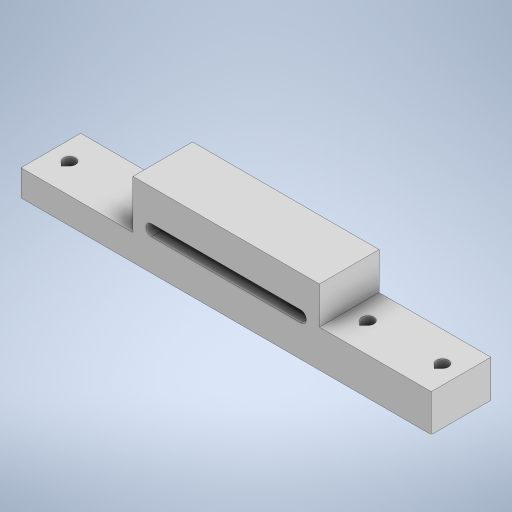
# Autodesk Inventor part: middle_hole
Saved by Autodesk Inventor 2023.1 (Build 271208000, 208)
## iProperties
Created: 2023-11-20
Part Number: middle_hole
Material: Všeobecné
Document SubType Name: Modeling
Designer: zavrel
Density: 1 g/cm^3
Appearance: Výchozí
Author: zavrel
Autodesk Inventor part; units mm, degrees
ref_plane "YZ Plane" through (0, 0, 0) normal (1, 0, 0) x (0, 1, 0)
ref_plane "XZ Plane" through (0, 0, 0) normal (0, 1, 0) x (-1, 0, 0)
ref_plane "XY Plane" through (0, 0, 0) normal (0, 0, 1) x (1, 0, 0)
sketch "Náčrt1" plane through (0, 0, 0) normal (0, 1, 0) x (-1, 0, 0)
  line L0 (0, 0) -> (110, 0)
  line L1 (110, 0) -> (110, -16)
  line L2 (110, -16) -> (0, -16)
  line L3 (0, -16) -> (0, 0)
  line L4 (55, -16) -> (55, 0) construction
  line L5 (110, -8) -> (0, -8) construction
  circle A0 centre (105, -8) radius 1.6
  circle A1 centre (85, -8) radius 1.6
  line L6 (105, -8) -> (105, -2.8731) construction
  line L7 (85, -8) -> (85, -2.8731) construction
  line L8 (105, -5.7373) -> (103.8686, -6.8686)
  line L9 (105, -5.7373) -> (106.1314, -6.8686)
  line L10 (85, -5.7373) -> (83.8686, -6.8686)
  line L11 (85, -5.7373) -> (86.1314, -6.8686)
  circle A2 centre (5, -8) radius 1.6
  circle A3 centre (25, -8) radius 1.6
  line L12 (5, -8) -> (5, -2.8731) construction
  line L13 (25, -8) -> (25, -2.8731) construction
  line L14 (5, -5.7373) -> (6.1314, -6.8686)
  line L15 (5, -5.7373) -> (3.8686, -6.8686)
  line L16 (25, -5.7373) -> (26.1314, -6.8686)
  line L17 (25, -5.7373) -> (23.8686, -6.8686)
  dimension "d0" = 16
  dimension "d1" = 110
  dimension "d4" = 3.2
  dimension "d6" = 25
  dimension "d7" = 5
  dimension "d49" = 90
  dimension "d54" = 90
  constraints: 36 end point, 10 symmetric about line, 4 centre point, 4 midpoint, 4 point on circle, 4 point on line, 2 parallel, 2 tangent, 2 vertical, 1 equal radius, 1 horizontal, 1 perpendicular, 2 other
  measures "d0" distance between parallel lines of L2 L0
  measures "d1" distance of L1.end L2.end
  measures "d4" diameter of A0
  measures "d6" distance from line of L1 L7.start
  measures "d7" distance from line of L1 L6.start
  measures "d49" angle of L9 L8
  measures "d54" angle of L11 L10
extrude "Vysunutí1" add sketch "Náčrt1" along normal blind 20
sketch "Sketch11" plane through (0, 20, 0) normal (0, 1, 0) x (1, 0, 0)
  line L0 (0, 16) -> (-110, 16) projected
  line L1 (-110, 16) -> (-110, 0) projected
  line L2 (-110, 0) -> (0, 0) projected
  line L3 (0, 0) -> (0, 16) projected
  arc A0 (-3.8686, 6.8686) -> (-6.1314, 6.8686) centre (-5, 8) ccw projected
  arc A1 (-23.8686, 6.8686) -> (-26.1314, 6.8686) centre (-25, 8) ccw projected
  arc A2 (-83.8686, 6.8686) -> (-86.1314, 6.8686) centre (-85, 8) ccw projected
  arc A3 (-103.8686, 6.8686) -> (-106.1314, 6.8686) centre (-105, 8) ccw projected
  line L4 (-30, 16) -> (-30, 0)
  line L5 (-110, 0) -> (0, 0) projected
  line L6 (-3.8686, 6.8686) -> (-5, 5.7373) projected
  line L7 (-5, 5.7373) -> (-6.1314, 6.8686) projected
  line L8 (-23.8686, 6.8686) -> (-25, 5.7373) projected
  line L9 (-25, 5.7373) -> (-26.1314, 6.8686) projected
  line L10 (-85, 5.7373) -> (-86.1314, 6.8686) projected
  line L11 (-83.8686, 6.8686) -> (-85, 5.7373) projected
  line L12 (-105, 5.7373) -> (-106.1314, 6.8686) projected
  line L13 (-103.8686, 6.8686) -> (-105, 5.7373) projected
  dimension "d55" = 30
  constraints: 2 end point, 2 point on line, 1 perpendicular
  measures "d55" distance between parallel lines of L3 L4
extrude "Extrusion9" cut sketch "Sketch11" against normal blind 10 contours L3 L2 L4 L0 | L6 L7 A0 | L8 L9 A1
sketch "Sketch12" plane through (0, 20, 0) normal (0, 1, 0) x (1, 0, 0)
  arc A0 (-103.8686, 6.8686) -> (-106.1314, 6.8686) centre (-105, 8) ccw projected
  arc A1 (-83.8686, 6.8686) -> (-86.1314, 6.8686) centre (-85, 8) ccw projected
  line L0 (-30, 0) -> (-30, 16) projected
  line L1 (-30, 16) -> (-110, 16) projected
  line L2 (-110, 16) -> (-110, 0) projected
  line L3 (-110, 0) -> (-30, 0) projected
  line L4 (0, 16) -> (-110, 16) projected
  line L5 (-80, 16) -> (-80, 0)
  line L6 (-110, 0) -> (0, 0) projected
  line L7 (-105, 5.7373) -> (-106.1314, 6.8686) projected
  line L8 (-103.8686, 6.8686) -> (-105, 5.7373) projected
  line L9 (-85, 5.7373) -> (-86.1314, 6.8686) projected
  line L10 (-83.8686, 6.8686) -> (-85, 5.7373) projected
  dimension "d58" = 30
  constraints: 2 end point, 2 point on line, 1 perpendicular
  measures "d58" distance between parallel lines of L5 L2
extrude "Extrusion10" cut sketch "Sketch12" against normal blind 13 contours L8 L7 A0 | L10 L9 A1 | L3 L2 L1 L5
sketch "Sketch14" plane through (0, 0, 0) normal (0, -1, 0) x (1, 0, 0)
  line L0 (0, -16) -> (-110, -16) projected
  line L1 (0, 0) -> (0, -16) projected
  line L2 (-110, 0) -> (0, 0) projected
  line L3 (-110, -16) -> (-110, 0) projected
  arc A0 (-6.1314, -6.8686) -> (-3.8686, -6.8686) centre (-5, -8) ccw projected
  arc A1 (-26.1314, -6.8686) -> (-23.8686, -6.8686) centre (-25, -8) ccw projected
  arc A2 (-86.1314, -6.8686) -> (-83.8686, -6.8686) centre (-85, -8) ccw projected
  arc A3 (-106.1314, -6.8686) -> (-103.8686, -6.8686) centre (-105, -8) ccw projected
  arc A4 (-106.1314, -6.8686) -> (-103.8686, -6.8686) centre (-105, -8) ccw projected
  line L4 (-105, -4.8246) -> (-102.25, -6.4123)
  line L5 (-102.25, -6.4123) -> (-102.25, -9.5877)
  line L6 (-102.25, -9.5877) -> (-105, -11.1754)
  line L7 (-105, -11.1754) -> (-107.75, -9.5877)
  line L8 (-107.75, -9.5877) -> (-107.75, -6.4123)
  line L9 (-107.75, -6.4123) -> (-105, -4.8246)
  line L10 (-5, -5.7373) -> (-6.1314, -6.8686) projected
  line L11 (-3.8686, -6.8686) -> (-5, -5.7373) projected
  line L12 (-25, -5.7373) -> (-26.1314, -6.8686) projected
  line L13 (-23.8686, -6.8686) -> (-25, -5.7373) projected
  line L14 (-85, -5.7373) -> (-86.1314, -6.8686) projected
  line L15 (-83.8686, -6.8686) -> (-85, -5.7373) projected
  line L16 (-105, -5.7373) -> (-106.1314, -6.8686) projected
  line L17 (-103.8686, -6.8686) -> (-105, -5.7373) projected
  line L18 (-110, -16) -> (-110, 0) projected
  line L19 (-85, -4.8246) -> (-82.25, -6.4123)
  line L20 (-82.25, -6.4123) -> (-82.25, -9.5877)
  line L21 (-82.25, -9.5877) -> (-85, -11.1754)
  line L22 (-85, -11.1754) -> (-87.75, -9.5877)
  line L23 (-87.75, -9.5877) -> (-87.75, -6.4123)
  line L24 (-87.75, -6.4123) -> (-85, -4.8246)
  line L25 (-25, -4.8246) -> (-22.25, -6.4123)
  line L26 (-22.25, -6.4123) -> (-22.25, -9.5877)
  line L27 (-22.25, -9.5877) -> (-25, -11.1754)
  line L28 (-25, -11.1754) -> (-27.75, -9.5877)
  line L29 (-27.75, -9.5877) -> (-27.75, -6.4123)
  line L30 (-27.75, -6.4123) -> (-25, -4.8246)
  line L31 (-5, -4.8246) -> (-2.25, -6.4123)
  line L32 (-2.25, -6.4123) -> (-2.25, -9.5877)
  line L33 (-2.25, -9.5877) -> (-5, -11.1754)
  line L34 (-5, -11.1754) -> (-7.75, -9.5877)
  line L35 (-7.75, -9.5877) -> (-7.75, -6.4123)
  line L36 (-7.75, -6.4123) -> (-5, -4.8246)
  point P0 (-85, -8)
  point P1 (-25, -8)
  dimension "d65" = 5.5
  dimension "d71" = 5.5
  dimension "d72" = 5.5
  dimension "d73" = 5.5
  constraints: 48 end point, 1 coincident, 1 parallel, 52 other
  measures "d65" distance between parallel lines of L5 L8
  measures "d71" distance between parallel lines of L20 L23
  measures "d72" distance between parallel lines of L26 L29
  measures "d73" distance between parallel lines of L32 L35
extrude "Extrusion12" cut sketch "Sketch14" against normal blind 2 contours L4 L5 L6 L7 L8 L9 | L19 L20 L21 L22 L23 L24 | L25 L26 L27 L28 L29 L30 | L31 L32 L33 L34 L35 L36
sketch "Sketch15" plane through (-110, 0, 0) normal (0, 0, 1) x (1, 0, 0)
  point P0 (110, 0)
sketch "Sketch16" plane through (-110, 0, 0) normal (0, 0, 1) x (1, 0, 0)
  line L0 (30, 7) -> (0, 7) projected
  line L1 (0, 0) -> (0, 7) projected
  line L2 (0, 0) -> (110, 0) projected
  line L3 (110, 0) -> (110, 10) projected
  line L4 (110, 10) -> (80, 10) projected
  line L5 (80, 10) -> (80, 20) projected
  line L6 (30, 20) -> (80, 20) projected
  line L7 (30, 20) -> (30, 7) projected
  line L8 (110, 0) -> (0, 0) construction
  line L9 (0, 0) -> (0, 20) construction
  line L10 (0, 20) -> (110, 20) construction
  line L11 (110, 20) -> (110, 0) construction
  line L12 (0, 20) -> (110, 0) construction
  line L13 (0, 0) -> (0, 7) construction
  line L14 (110, 20) -> (0, 0) construction
  line L15 (35, 10) -> (75, 10) construction
  line L16 (35, 8.5) -> (75, 8.5)
  line L17 (75, 11.5) -> (35, 11.5)
  arc A0 (35, 11.5) -> (35, 8.5) centre (35, 10) ccw
  arc A1 (75, 8.5) -> (75, 11.5) centre (75, 10) ccw
  point P0 (55, 10)
  dimension "d74" = 3
  dimension "d75" = 40
  constraints: 20 end point, 4 point on circle, 4 tangent, 3 parallel, 2 centre point, 2 horizontal, 2 midpoint, 1 perpendicular
  measures "d74" distance between parallel lines of L16 L17
  measures "d75" distance of L15.end L15.start
extrude "Extrusion13" cut sketch "Sketch16" against normal through all contours A0 L17 A1 L16
